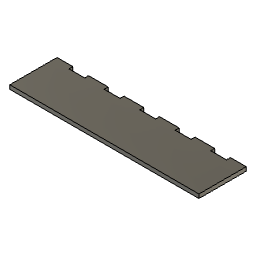
side v1 (Autodesk Fusion 360 design; units mm, degrees)
Autodesk Fusion 360 part; units mm, degrees
sketch "Sketch1" plane through (0, 0, 0) normal (0, 0, 1) x (1, 0, 0)
  line L0 (-152.4, 0) -> (152.4, 0)
  line L1 (152.4, 0) -> (152.4, -76.2)
  line L2 (152.4, -76.2) -> (-152.4, -76.2)
  line L3 (-152.4, -76.2) -> (-152.4, 0)
  dimension "d1" = 304.8
  dimension "d2" = 76.2
  dimension "d3" = 152.4
  constraint horizontal L0
  constraint vertical L1
  constraint horizontal L2
  constraint vertical L3
  constraint horizontal origin L0.start
  measures "d1" distance of L0.start L0.end
  measures "d2" distance of L0.start L2.end
  measures "d3" horizontal distance of origin L0.start
extrude "Extrude1" add sketch "Sketch1" along normal blind 6.35
sketch "Sketch2" plane through (0, 0, 6.35) normal (0, 0, 1) x (-1, 0, 0)
  line L0 (152.4, 76.2) -> (-152.4, 76.2)
  line L1 (-152.4, 76.2) -> (-152.4, 0)
  line L2 (-152.4, 0) -> (152.4, 0)
  line L3 (152.4, 0) -> (152.4, 76.2)
  line L4 (127, 0) -> (101.6, 0)
  line L5 (101.6, 0) -> (101.6, 6.35)
  line L6 (101.6, 6.35) -> (127, 6.35)
  line L7 (127, 6.35) -> (127, 0)
  dimension "d6" = 6.35
  dimension "d7" = 25.4
  dimension "d8" = 25.4
  constraint horizontal L4
  constraint vertical L5
  constraint horizontal L6
  constraint vertical L7
  constraint coincident L2 L4.start
  measures "d6" distance of L4.start L6.end
  measures "d7" distance of L4.start L4.end
  measures "d8" distance of L2.end L4.start
extrude "Extrude2" cut sketch "Sketch2" against normal through all contours L2 L4 L5 L6 L7
pattern_path "PathPattern1" count 5 spacing 57.15 from (-101.6, 0, 6.35) along 1 edges at (25.4, 0, 6.35) of "Extrude2"
